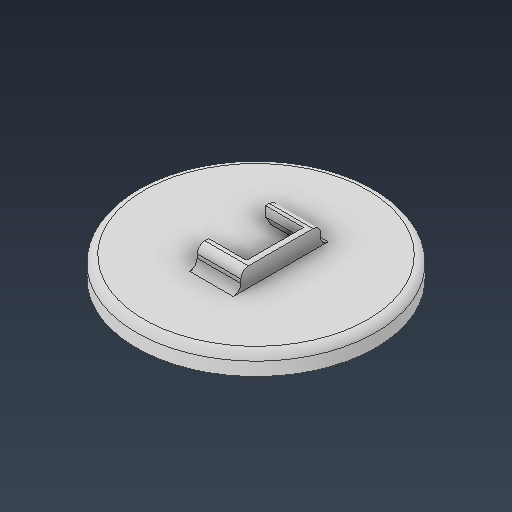
# Autodesk Inventor part: magnet
Saved by Autodesk Inventor 2025.3 (Build 293356000, 356)
## iProperties
Created: 2025-11-24
Part Number: magnet
Material: 一般
Document SubType Name: Modeling
Designer: 陳泓任
Density: 1 g/cm^3
Appearance: 預設
Author: 陳泓任
Autodesk Inventor part; units mm, degrees
ref_plane "YZ Plane" through (0, 0, 0) normal (1, 0, 0) x (0, 1, 0)
ref_plane "XZ Plane" through (0, 0, 0) normal (0, 1, 0) x (-1, 0, 0)
ref_plane "XY Plane" through (0, 0, 0) normal (0, 0, 1) x (1, 0, 0)
sketch "草圖1" plane through (0, 0, 0) normal (0, 1, 0) x (-1, 0, 0)
  arc A0 (-8.4452, 27.7431) -> (8.4452, 27.7431) centre (0, 0) ccw
  arc A1 (-5.9383, 20.6637) -> (5.9383, 20.6637) centre (0, 0) ccw
  line L0 (-30.6072, 0) -> (30.6072, 0) construction
  line L1 (0, 30.3417) -> (0, -30.3417) construction
  line L2 (0, 0) -> (9.6804, 27.3366) construction
  line L3 (0, 0) -> (-9.6804, 27.3366) construction
  line L4 (-9.0128, 25.4513) -> (-7.6108, 21.4922)
  line L5 (9.0128, 25.4513) -> (7.6108, 21.4922)
  line L6 (5.9383, 20.6637) -> (8.4452, 27.7431)
  line L7 (-5.9383, 20.6637) -> (-8.4452, 27.7431)
  arc A2 (26.9896, 0.75) -> (9.0128, 25.4513) centre (0, 0) ccw
  arc A3 (-9.0128, 25.4513) -> (-26.9896, 0.75) centre (0, 0) ccw
  arc A4 (22.7877, 0.75) -> (7.6108, 21.4922) centre (0, 0) ccw
  arc A5 (-7.6108, 21.4922) -> (-22.7877, 0.75) centre (0, 0) ccw
  line L8 (0, 0) -> (11.7954, -26.4928) construction
  line L9 (0, 0) -> (-11.7954, -26.4928) construction
  line L10 (8.7448, -19.6412) -> (11.7954, -26.4928) construction
  line L11 (8.676, -21.0847) -> (10.3849, -24.923)
  line L12 (9.8636, -20.556) -> (11.5725, -24.3942)
  line L13 (-8.676, -21.0847) -> (-10.3849, -24.923)
  line L14 (-9.8636, -20.556) -> (-11.5725, -24.3942)
  arc A6 (-22.7877, -0.75) -> (-9.8636, -20.556) centre (0, 0) ccw
  arc A7 (-26.9896, -0.75) -> (-11.5725, -24.3942) centre (0, 0) ccw
  arc A8 (-8.676, -21.0847) -> (8.676, -21.0847) centre (0, 0) ccw
  arc A9 (9.8636, -20.556) -> (22.7877, -0.75) centre (0, 0) ccw
  arc A10 (-10.3849, -24.923) -> (10.3849, -24.923) centre (0, 0) ccw
  arc A11 (11.5725, -24.3942) -> (26.9896, -0.75) centre (0, 0) ccw
  arc A12 (22.7877, -0.75) -> (22.7877, 0.75) centre (0, 0) ccw
  arc A13 (26.9896, -0.75) -> (26.9896, 0.75) centre (0, 0) ccw
  arc A14 (10.3849, -24.923) -> (11.5725, -24.3942) centre (0, 0) ccw
  arc A15 (8.676, -21.0847) -> (9.8636, -20.556) centre (0, 0) ccw
  arc A16 (-9.8636, -20.556) -> (-8.676, -21.0847) centre (0, 0) ccw
  arc A17 (-11.5725, -24.3942) -> (-10.3849, -24.923) centre (0, 0) ccw
  arc A18 (-22.7877, 0.75) -> (-22.7877, -0.75) centre (0, 0) ccw
  arc A19 (-26.9896, 0.75) -> (-26.9896, -0.75) centre (0, 0) ccw
  line L15 (0, 0) -> (33.3815, 4.6716) construction
  line L16 (5.9383, 20.6637) -> (0, 0) construction
  line L17 (26.7531, 3.643) -> (22.5936, 3.0609)
  line L18 (26.8975, 2.3505) -> (22.7314, 1.7675)
  line L19 (-26.7531, 3.643) -> (-22.5936, 3.0609)
  line L20 (-26.8975, 2.3505) -> (-22.7314, 1.7675)
  dimension "d0" = 58
  dimension "d1" = 43
  dimension "d8" = 39
  dimension "d9" = 1.3
  dimension "d10" = 22.8
  dimension "d12" = 48
  dimension "d13" = 1.3
  dimension "d14" = 27
  dimension "d15" = 1.3
  dimension "d28" = 66
  dimension "d30" = 1.3
  dimension "d31" = 0.1
  constraints: 48 point on circle, 42 end point, 20 centre point, 14 symmetric about line, 10 concentric, 4 coincident, 4 parallel, 3 collinear, 2 midpoint, 1 horizontal, 1 point on line, 1 vertical, 2 other
  measures "d0" diameter of A0
  measures "d1" diameter of A1
  measures "d8" angle of L2 L3
  measures "d9" distance between parallel lines of L6 L5
  measures "d10" radius of A4
  measures "d12" angle of L9 L8
  measures "d13" distance between parallel lines of L11 L12
  measures "d14" radius of A11
  measures "d15" distance between parallel lines of L14 L13
  measures "d28" angle of L16 L15
  measures "d30" distance between parallel lines of L17 L18
  measures "d31" distance from line of L15 L17.end
extrude "支撐處(低一點)" add sketch "草圖1" along normal blind 1.54 contours L19 A5 L20 A3 | L14 A16 L13 A17 | L11 A15 L12 A14 | L18 A4 L17 A2
extrude "框架" add sketch "草圖1" along normal blind 2
sketch "草圖2" plane through (0, 0, 0) normal (0, -1, 0) x (1, 0, 0)
  circle A0 centre (0, 0) radius 31.5
  dimension "d18" = 63
  constraints: 1 centre point, 1 coincident
  measures "d18" diameter of A0
extrude "底盤" add sketch "草圖2" along normal blind 0.5
sketch "草圖6" plane through (0, 0, 0) normal (0, 1, 0) x (1, 0, 0)
  arc A0 (5.9383, -20.6637) -> (-5.9383, -20.6637) centre (0, 0) ccw projected
  line L0 (-8.4452, -27.7431) -> (-5.9383, -20.6637) projected
  line L1 (5.9383, -20.6637) -> (8.4452, -27.7431) projected
  arc A1 (-8.4452, -27.7431) -> (8.4452, -27.7431) centre (0, 0) ccw
  arc A2 (8.4452, -27.7431) -> (-8.4452, -27.7431) centre (0, 0) ccw projected
  constraints: 2 point on circle, 1 centre point, 1 concentric
extrude "填中空" add sketch "草圖6" along normal blind 2.5 contours L1 A1 L0 A0
sketch "草圖3" plane through (0, 0, 0) normal (1, 0, 0) x (0, 1, 0)
  line L0 (0, -31.5) -> (5, -31.5)
  line L1 (5, -31.5) -> (5, 0)
  line L2 (0, -31.5) -> (-0.5, -31.5) projected
  line L3 (10.6669, 0) -> (-5.2502, 0)
  line L4 (0, 31.5) -> (0, -31.5) projected
  line L5 (0, -29) -> (0, -31.5)
  line L6 (2.5, 0) -> (2.5, -29)
  line L7 (2.5, -29) -> (0, -29)
  line L8 (2, -29) -> (2, 27.7431) projected
  line L9 (5, 0) -> (2.5719, 0)
  point P0 (0, 0)
  point P1 (2, 0)
  point P2 (0, 0)
  dimension "d43" = 0.5
  dimension "d44" = 2.5
  constraints: 14 end point, 2 collinear, 2 horizontal, 2 point on line, 1 perpendicular
  measures "d43" distance between parallel lines of L8 L6
  measures "d44" distance between parallel lines of L6 L1
revolve "蓋子" add sketch "草圖3" angle 360 about axis through (0, 10.6669, 0) along (0, -1, 0) contours L4 L7 L6 L3 L1 L0
fillet "圓角2" radius 2 1 edges at (0, 5, 31.5)
sketch "草圖4" plane through (0, 0, 0) normal (1, 0, 0) x (0, 1, 0)
  line L0 (10, 10.5) -> (5, 10.5)
  line L1 (5, 29.5) -> (5, -29.5) projected
  line L2 (5, 8.9) -> (7.4249, 7.5)
  line L3 (7.4249, 7.5) -> (10, 7.5)
  line L4 (10, 7.5) -> (10, 10.5)
  line L5 (5, 10.5) -> (5, 8.9)
  line L6 (15.2315, 0) -> (-3.1716, 0)
  line L7 (10, -10.5) -> (5, -10.5)
  line L8 (5, -8.9) -> (7.4249, -7.5)
  line L9 (7.4249, -7.5) -> (10, -7.5)
  line L10 (10, -7.5) -> (10, -10.5)
  line L11 (5, -10.5) -> (5, -8.9)
  point P0 (0, 0)
  dimension "d35" = 15
  dimension "d36" = 3
  dimension "d37" = 60
  dimension "d38" = 5
  dimension "d39" = 1.6
  constraints: 22 end point, 5 symmetric about line, 3 horizontal, 2 point on line, 1 collinear, 1 parallel, 1 perpendicular
  measures "d35" diameter of L3 L6
  measures "d36" distance of L3.end L0.start
  measures "d37" angle of L1 L2
  measures "d38" distance of L0.start L0.end
  measures "d39" distance of L0.end L2.start
extrude "擠出4" add sketch "草圖4" along normal mid plane 10
fillet "圓角3" radius 2 4 edges at (0, 5, 10.5) (0, 5, -10.5) (0, 10, -10.5) (0, 10, 10.5)
sketch "草圖5" plane through (5, 0, 0) normal (1, 0, 0) x (0, 0, -1)
  arc A0 (-8.5, 10) -> (-10.5, 8) centre (-8.5, 8) ccw projected
  line L0 (-8.9, 5) -> (-7.5, 7.4249) projected
  line L1 (-7.5, 7.4249) -> (-7.5, 10) projected
  line L2 (-7.5, 10) -> (-8.5, 10) projected
  arc A1 (10.5, 8) -> (8.5, 10) centre (8.5, 8) ccw projected
  line L3 (8.5, 10) -> (7.5, 10) projected
  line L4 (7.5, 10) -> (7.5, 7.4249) projected
  line L5 (7.5, 7.4249) -> (8.9, 5) projected
  line L6 (-7.5, 10) -> (7.5, 10)
  line L7 (-8.9, 5) -> (8.9, 5)
  line L8 (12.5, 5) -> (8.9, 5) projected
  arc A2 (10.5, 7) -> (12.5, 5) centre (12.5, 7) ccw projected
  arc A3 (-12.5, 5) -> (-10.5, 7) centre (-12.5, 7) ccw projected
  line L9 (-8.9, 5) -> (-12.5, 5) projected
  line L10 (10.5, 7) -> (10.5, 8) projected
  line L11 (-10.5, 8) -> (-10.5, 7) projected
  point P0 (0, 0)
  constraints: 4 end point, 1 horizontal
extrude "擠出5" add sketch "草圖5" along normal blind 1.5
